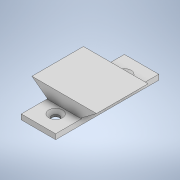
# Autodesk Inventor part: DoveTail_Joint_1
Saved by Autodesk Inventor 2022.3 (Build 263350000, 350)
## iProperties
Created: 2023-05-19
Part Number: DoveTail_Joint_1
Material: Generic
Document SubType Name: Modeling
Designer: Manuel Hueso Béjar
Density: 1 g/cm^3
Appearance: Default
Author: Manuel Hueso Béjar
Autodesk Inventor part; units mm, degrees
ref_plane "YZ Plane" through (0, 0, 0) normal (1, 0, 0) x (0, 1, 0)
ref_plane "XZ Plane" through (0, 0, 0) normal (0, 1, 0) x (-1, 0, 0)
ref_plane "XY Plane" through (0, 0, 0) normal (0, 0, 1) x (1, 0, 0)
sketch "Sketch1" plane through (0, 0, 0) normal (0, 1, 0) x (-1, 0, 0)
  line L0 (-5, 15) -> (5, 15)
  line L1 (5, 15) -> (5, -15)
  line L2 (5, -15) -> (-5, -15)
  line L3 (-5, -15) -> (-5, 15)
  line L4 (-5, 15) -> (5, -15) construction
  line L5 (5, 15) -> (-5, -15) construction
  point P0 (0, 0)
  dimension "d0" = 10
  dimension "d1" = 30
  constraints: 12 end point, 2 midpoint, 2 parallel, 1 horizontal, 1 perpendicular
  measures "d0" distance of L1.end L2.end
  measures "d1" distance of L0.end L1.end
extrude "Extrusion1" add sketch "Sketch1" along normal blind 1.5
sketch "Sketch2" plane through (0, 1.5, 0) normal (0, 1, 0) x (1, 0, 0)
  line L0 (0, 0) -> (0, 10)
  line L1 (0, 10) -> (0, -10)
  dimension "d4" = 10
  dimension "d5" = 20
  constraints: 4 end point, 1 point on line, 1 vertical
  measures "d4" distance of L0.start L0.end
  measures "d5" distance of L0.end L1.end
hole "Hole1" at (0, 1.5, 10) at (0, 1.5, -10) direction (0, -1, 0) diameter 2.2 end through all countersink diameter 4 countersink angle 90
sketch "Sketch3" plane through (0, 0, 0) normal (0, 0, 1) x (1, 0, 0)
  line L0 (-10, -2.25) -> (10, -2.25)
  line L1 (10, -2.25) -> (10, 5.25)
  line L2 (10, 5.25) -> (-10, 5.25)
  line L3 (-10, 5.25) -> (-10, -2.25)
  line L4 (5, 1.5) -> (-5, 1.5) projected
  line L5 (-10, -2.25) -> (10, 5.25) construction
  line L6 (10, -2.25) -> (-10, 5.25) construction
  line L7 (-10, 5.25) -> (-5, 1.5)
  line L8 (5, 1.5) -> (10, 5.25)
  line L9 (-5, 1.5) -> (5, 1.5)
  point P0 (0, 0)
  point P1 (0, 1.5)
  dimension "d13" = 20
  dimension "d14" = 7.5
  constraints: 18 end point, 3 midpoint, 2 parallel, 1 horizontal, 1 perpendicular
  measures "d13" distance of L2.end L1.end
  measures "d14" distance of L1.end L0.end
extrude "Extrusion2" add sketch "Sketch3" along normal blind 7.5 and the other way blind 7.5 contours L2 L8 L4 L7
thicken "Thicken1" operation add thickness 0.2 both sides no extend neighbours yes toward (0, -1, 0) faces at (-3.3333, 5.25, 2.5)
thicken "Thicken2" operation add thickness 0.2 both sides no extend neighbours yes toward (-0.6, 0.8, 0) faces at (6.5778, 2.6833, -2.5)
thicken "Thicken3" operation add thickness 0.2 both sides no extend neighbours yes toward (0.6, 0.8, 0) faces at (-6.5778, 2.6833, 2.5)
body "Solid1"
